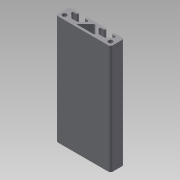
# Autodesk Inventor part: 25-5013
Saved by Autodesk Inventor 2013 (Build 170138000, 138)
## iProperties
Created: 2014-04-23
Part Number: 25-5013
Material: Generic
Document SubType Name: Modeling
Designer: Ross Bowman
Density: 1 g/cm^3
Engineer: Ross Bowman
Catalog Web Link: 8020.net
Vendor: 80/20 Inc.
Company: 80/20 Inc.
Author: Ross Bowman
Keywords: 80/20 , 8020 , T-Slot , Extrusion
Material: 6105-T5 Aluminum
Autodesk Inventor part; units mm, degrees
ref_plane "YZ Plane" through (0, 0, 0) normal (1, 0, 0) x (0, 1, 0)
ref_plane "XZ Plane" through (0, 0, 0) normal (0, 1, 0) x (-1, 0, 0)
ref_plane "XY Plane" through (0, 0, 0) normal (0, 0, 1) x (1, 0, 0)
sketch "Sketch1" plane through (0, 0, 0) normal (0, 0, 1) x (1, 0, 0)
  arc A0 (-0.4146, 4.1159) -> (-0.7739, 3.967) centre (-0.4146, 3.6077) ccw
  line L0 (0.4146, 4.1159) -> (-0.4146, 4.1159)
  arc A1 (0.7154, 4.0255) -> (0.4146, 4.1159) centre (0.426, 3.6079) ccw
  line L1 (7.9894, -3.2484) -> (0.7154, 4.0255)
  arc A2 (7.63, -4.1159) -> (7.9894, -3.2484) centre (7.63, -3.6077) ccw
  line L2 (-7.63, -4.1159) -> (7.63, -4.1159)
  arc A3 (-7.9894, -3.2484) -> (-7.63, -4.1159) centre (-7.63, -3.6077) ccw
  line L3 (-0.7739, 3.967) -> (-7.9894, -3.2484)
  circle A4 centre (-21.0112, -2.2612) radius 2
  circle A5 centre (21.0112, -2.2612) radius 2
  arc A6 (-23.0183, 6.25) -> (-25, 4.2683) centre (-23.0183, 4.2683) ccw
  line L4 (-25, 4.2683) -> (-25, -4.2683)
  arc A7 (-25, -4.2683) -> (-23.0183, -6.25) centre (-23.0183, -4.2683) ccw
  line L5 (-23.0183, -6.25) -> (23.0183, -6.25)
  arc A8 (23.0183, -6.25) -> (25, -4.2683) centre (23.0183, -4.2683) ccw
  line L6 (25, -4.2683) -> (25, 4.2683)
  arc A9 (25, 4.2683) -> (23.0183, 6.25) centre (23.0183, 4.2683) ccw
  line L7 (23.0183, 6.25) -> (16.82, 6.25)
  arc A10 (16.82, 6.25) -> (16.82, 4.11) centre (16.82, 5.18) ccw
  line L8 (16.82, 4.11) -> (18.9356, 4.11)
  arc A11 (19.6349, 2.4086) -> (18.9356, 4.11) centre (18.9356, 3.1156) ccw
  line L9 (19.6349, 2.4086) -> (16.275, -0.9151)
  arc A12 (14.0005, -1.85) -> (16.275, -0.9151) centre (14.0005, 1.3841) ccw
  line L10 (14.0005, -1.85) -> (10.9995, -1.85)
  arc A13 (8.725, -0.9151) -> (10.9995, -1.85) centre (10.9995, 1.3841) ccw
  line L11 (8.725, -0.9151) -> (5.3651, 2.4086)
  arc A14 (6.0644, 4.11) -> (5.3651, 2.4086) centre (6.0644, 3.1156) ccw
  line L12 (6.0644, 4.11) -> (8.18, 4.11)
  arc A15 (8.18, 4.11) -> (8.18, 6.25) centre (8.18, 5.18) ccw
  line L13 (8.18, 6.25) -> (-8.18, 6.25)
  arc A16 (-8.18, 6.25) -> (-8.18, 4.11) centre (-8.18, 5.18) ccw
  line L14 (-8.18, 4.11) -> (-6.0644, 4.11)
  arc A17 (-5.3651, 2.4086) -> (-6.0644, 4.11) centre (-6.0644, 3.1156) ccw
  line L15 (-5.3651, 2.4086) -> (-8.725, -0.9151)
  arc A18 (-10.9995, -1.85) -> (-8.725, -0.9151) centre (-10.9995, 1.3841) ccw
  line L16 (-10.9995, -1.85) -> (-14.0005, -1.85)
  arc A19 (-16.275, -0.9151) -> (-14.0005, -1.85) centre (-14.0005, 1.3841) ccw
  line L17 (-16.275, -0.9151) -> (-19.6349, 2.4086)
  arc A20 (-18.9356, 4.11) -> (-19.6349, 2.4086) centre (-18.9356, 3.1156) ccw
  line L18 (-18.9356, 4.11) -> (-16.82, 4.11)
  arc A21 (-16.82, 4.11) -> (-16.82, 6.25) centre (-16.82, 5.18) ccw
  line L19 (-16.82, 6.25) -> (-23.0183, 6.25)
  point P0 (0, 0)
  constraints: 40 end point, 40 point on circle, 22 centre point
extrude "Extrusion1" add sketch "Sketch1" against normal blind 100
body "Solid1"
